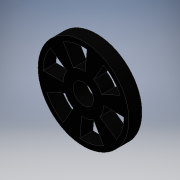
# Autodesk Inventor part: Brushless Motor Case
Saved by Autodesk Inventor 2016 (Build 200138000, 138)
## iProperties
Created: 2015-12-30
Part Number: Brushless Motor Case
Material: Generic
Document SubType Name: Modeling
Designer: jonathan
Density: 1 g/cm^3
Appearance: Fine Textured - Black
Author: jonathan
Autodesk Inventor part; units mm, degrees
ref_plane "YZ Plane" through (0, 0, 0) normal (1, 0, 0) x (0, 1, 0)
ref_plane "XZ Plane" through (0, 0, 0) normal (0, 1, 0) x (-1, 0, 0)
ref_plane "XY Plane" through (0, 0, 0) normal (0, 0, 1) x (1, 0, 0)
sketch "Sketch1" plane through (0, 0, 0) normal (0, 1, 0) x (-1, 0, 0)
  circle A0 centre (0, 0) radius 45
  dimension "d0" = 90
  constraints: 1 centre point, 1 coincident
  measures "d0" diameter of A0
extrude "Extrusion1" add sketch "Sketch1" along normal blind 13
sketch "Sketch2" plane through (0, 0, 0) normal (0, 1, 0) x (-1, 0, 0)
  circle A0 centre (0, 0) radius 10
  line L0 (0, 0) -> (-40, 0)
  line L1 (0, 0) -> (-32.7661, -22.9431)
  arc A1 (-20, 0) -> (-16.383, -11.4715) centre (0, 0) ccw
  arc A2 (-40, 0) -> (-32.7661, -22.9431) centre (0, 0) ccw
  dimension "d3" = 20
  dimension "d5" = 35
  dimension "d16" = 40
  constraints: 4 coincident, 4 end point, 4 point on circle, 3 centre point, 2 midpoint, 1 horizontal
  measures "d3" diameter of A0
  measures "d5" angle of L1 L0
  measures "d16" distance of L0.start L0.end
extrude "Extrusion2" cut sketch "Sketch2" along normal blind 13 contours A0 L1 L0 | L0 L1 A0 | A1 L1 A2 L0
pattern_circular "Circular Pattern1" count 6 over 360 about axis through (0, 0, 0) along (0, 1, 0) of "Extrusion2"
body "Solid1"
